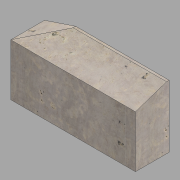
# Autodesk Inventor part: Straight_C21
Saved by Autodesk Inventor 2022.1 (Build 261234020, 234B)
## iProperties
Created: 2021-12-03
Part Number: Straight_C21
Material: Limestone
Document SubType Name: Modeling
Designer: awelt
Density: 2.6 g/cm^3
Appearance: Kasota Gray
Author: awelt
Autodesk Inventor part; units mm, degrees
ref_plane "YZ Plane" through (0, 0, 0) normal (1, 0, 0) x (0, 1, 0)
ref_plane "XZ Plane" through (0, 0, 0) normal (0, 1, 0) x (-1, 0, 0)
ref_plane "XY Plane" through (0, 0, 0) normal (0, 0, 1) x (1, 0, 0)
sketch "Sketch1" plane through (0, 0, 0) normal (0, 1, 0) x (-1, 0, 0)
  line L0 (-304.8, -82.55) -> (304.8, -82.55)
  line L1 (304.8, -82.55) -> (304.8, 82.55)
  line L2 (304.8, 82.55) -> (-304.8, 82.55)
  line L3 (-304.8, 82.55) -> (-304.8, -82.55)
  line L4 (-304.8, -82.55) -> (304.8, 82.55) construction
  line L5 (304.8, -82.55) -> (-304.8, 82.55) construction
  point P0 (0, 0)
  dimension "d0" = 609.6
  dimension "d1" = 165.1
  constraints: 12 end point, 2 midpoint, 2 parallel, 1 horizontal, 1 perpendicular
  measures "d0" distance of L2.end L1.end
  measures "d1" distance of L1.end L0.end
extrude "Extrusion1" add sketch "Sketch1" along normal blind 304.8
sketch "Sketch2" plane through (304.8, 0, 82.55) normal (1, 0, 0) x (0, 0, -1)
  line L0 (165.1, 304.8) -> (0, 304.8) projected
  line L1 (0, 0) -> (0, 304.8) projected
  line L2 (152.4, 304.8) -> (0, 254)
  line L3 (0, 304.8) -> (0, 254)
  line L4 (0, 304.8) -> (152.4, 304.8)
  point P0 (82.55, 0)
  dimension "d4" = 50.8
  dimension "d5" = 152.4
  constraints: 6 end point, 2 point on line, 1 collinear, 1 vertical
  measures "d4" distance of L2.end L0.end
  measures "d5" distance of L2.start L0.end
extrude "Extrusion2" cut sketch "Sketch2" against normal through all
sketch "Sketch3" plane through (304.8, 0, -82.55) normal (0, 0, -1) x (-1, 0, 0)
  line L0 (0, 304.8) -> (609.6, 304.8) projected
  line L1 (609.6, 0) -> (609.6, 304.8) projected
  line L2 (457.2, 304.8) -> (609.6, 254)
  line L3 (609.6, 304.8) -> (609.6, 254)
  line L4 (609.6, 304.8) -> (457.2, 304.8)
  point P0 (304.8, 0)
  dimension "d8" = 152.4
  dimension "d9" = 50.8
  constraints: 6 end point, 2 collinear, 2 point on line
  measures "d8" distance of L2.start L0.end
  measures "d9" distance of L2.end L0.end
extrude "Extrusion3" cut sketch "Sketch3" against normal through all
body "Solid1"
